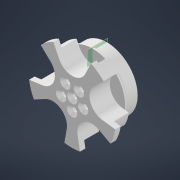
# Autodesk Inventor part: tire cap
Saved by Autodesk Inventor 2022 (Build 260153000, 153)
## iProperties
Created: 2023-02-07
Part Number: tire cap
Material: Типовые
Document SubType Name: Modeling
Designer: akapu
Density: 1 g/cm^3
Appearance: По умолчанию
Author: akapu
Autodesk Inventor part; units mm, degrees
ref_plane "YZ Plane" through (0, 0, 0) normal (1, 0, 0) x (0, 1, 0)
ref_plane "XZ Plane" through (0, 0, 0) normal (0, 1, 0) x (-1, 0, 0)
sketch "Эскиз1" plane through (0, 0, 0) normal (0, 0, 1) x (1, 0, 0)
  circle A0 centre (-27.3933, 9.5988) radius 21.25 projected
  circle A1 centre (-27.3933, 9.5988) radius 18.75 projected
  point P0 (0, 0)
ref_plane "РабПлоскость1" through (-34.9651, 34.6315, 13) normal (0, 0, 1) x (1, 0, 0)
extrude "Выдавливание1" add sketch "Эскиз1" along normal up to surface (13 mm away) contours A0 | A1
ref_plane "РабПлоскость3" through (-27.3933, 9.5988, 13) normal (-1, 0, 0) x (0, -1, 0)
sketch "Эскиз3" plane through (-27.3933, 9.5988, 13) normal (-1, 0, 0) x (0, -1, 0)
  line L0 (-22.45, -4.27) -> (-21.25, -5.47)
  line L1 (-22.45, -3.07) -> (-22.45, -4.27)
  line L2 (30, -3.07) -> (-30, -3.07) projected
  line L3 (30, -3.07) -> (-30, -3.07) projected
  line L4 (-21.25, 0) -> (21.25, 0) projected
  line L5 (-21.25, 0) -> (-30, 0)
  line L6 (-30, 0) -> (-30, -3.07)
  line L7 (-30, -3.07) -> (-21.25, -3.07)
  line L8 (-21.25, -3.07) -> (-21.25, 0)
  line L9 (0, 0) -> (0, -13)
  line L10 (21.25, -13) -> (-21.25, -13) projected
  line L11 (-21.25, -13) -> (-21.25, 0) projected
  line L12 (0, 0) -> (-30, 0)
  line L13 (-30, 0) -> (-30, 11)
  line L14 (-30, 11) -> (0, 11)
  line L15 (0, 11) -> (0, 0)
  line L16 (-25.52, 6.93) -> (-25.52, -23)
  line L17 (-25.32, 6.93) -> (-25.32, -23)
  line L18 (-25.32, 6.93) -> (-25.32, 11)
  line L19 (-25.32, 6.93) -> (-30, 6.93)
  line L20 (-25.32, 7.23) -> (-30, 7.23)
  point P0 (9.5988, -13)
  point P1 (-21.25, -3.07)
  point P2 (-25.32, -3.07)
  dimension "d21" = 11
  dimension "d25" = 0.2
  dimension "d26" = 0.3
  constraints: 32 end point, 6 parallel, 4 perpendicular, 2 horizontal, 2 midpoint, 2 point on line, 2 vertical, 6 other
  measures "d21" distance of L12.end L13.end
  measures "d25" distance between parallel lines of L16 L17
  measures "d26" distance between parallel lines of L19 L20
revolve "Вращение1" add sketch "Эскиз3" angle 360 about axis through (-27.3933, 9.5988, 13) along (0, 0, -1) contours L1 L2 L11 L0 | L2 L17 L5 L8 | L5 L17 L18 L14 L15 L4 | L20 L13 L14 L18
sketch "Эскиз5" plane through (-27.3933, 9.5988, 24) normal (0, 0, 1) x (1, 0, 0)
  circle A0 centre (0, 0) radius 22.45 projected
  line L0 (-30.0943, 4.3007) -> (-34.526, 5.7406) projected
  arc A1 (-34.526, 5.7406) -> (-24.5579, -24.9382) centre (0, 0) ccw projected
  line L1 (-24.5579, -24.9382) -> (-21.8189, -21.1683) projected
  arc A2 (-21.8189, -21.1683) -> (-13.3898, -27.2924) centre (0, 0) ccw projected
  line L2 (-13.3898, -27.2924) -> (-16.1288, -31.0622) projected
  arc A3 (-16.1288, -31.0622) -> (16.1288, -31.0622) centre (0, 0) ccw projected
  line L3 (16.1288, -31.0622) -> (13.3898, -27.2924) projected
  arc A4 (13.3898, -27.2924) -> (21.8189, -21.1683) centre (0, 0) ccw projected
  line L4 (21.8189, -21.1683) -> (24.5579, -24.9382) projected
  arc A5 (24.5579, -24.9382) -> (34.526, 5.7406) centre (0, 0) ccw projected
  line L5 (34.526, 5.7406) -> (30.0943, 4.3007) projected
  arc A6 (30.0943, 4.3007) -> (26.8746, 14.2096) centre (0, 0) ccw projected
  line L6 (26.8746, 14.2096) -> (31.3064, 15.6496) projected
  arc A7 (31.3064, 15.6496) -> (5.2094, 34.6101) centre (0, 0) ccw projected
  line L7 (5.2094, 34.6101) -> (5.2094, 29.9503) projected
  arc A8 (5.2094, 29.9503) -> (-5.2094, 29.9503) centre (0, 0) ccw projected
  line L8 (-5.2094, 29.9503) -> (-5.2094, 34.6101) projected
  arc A9 (-5.2094, 34.6101) -> (-31.3064, 15.6496) centre (0, 0) ccw projected
  line L9 (-31.3064, 15.6496) -> (-26.8746, 14.2096) projected
  arc A10 (-26.8746, 14.2096) -> (-30.0943, 4.3007) centre (0, 0) ccw projected
  line L10 (3.8059, -20.9064) -> (6.2685, -34.4341) projected
  line L11 (18.7071, -10.0801) -> (30.8117, -16.6024) projected
  line L12 (21.0593, -2.8408) -> (34.6858, -4.679) projected
  line L13 (15.3675, 14.6766) -> (25.3112, 24.1732) projected
  line L14 (9.2094, 19.1507) -> (15.1685, 31.5423) projected
  line L15 (-9.2094, 19.1507) -> (-15.1685, 31.5423) projected
  line L16 (-15.3675, 14.6766) -> (-25.3112, 24.1732) projected
  line L17 (-21.0593, -2.8408) -> (-34.6858, -4.679) projected
  line L18 (-18.7071, -10.0801) -> (-30.8117, -16.6024) projected
  line L19 (-3.8059, -20.9064) -> (-6.2685, -34.4341) projected
  circle A11 centre (0, 0) radius 21.25 projected
  line L20 (-9.2094, 19.1507) -> (-9.0121, 18.7403)
  line L21 (9.0121, 18.7403) -> (9.2094, 19.1507)
  line L22 (15.3675, 14.6766) -> (15.0382, 14.3621)
  line L23 (21.0593, -2.8408) -> (20.608, -2.7799)
  line L24 (18.7071, -10.0801) -> (18.3062, -9.864)
  line L25 (3.8059, -20.9064) -> (3.7243, -20.4584)
  line L26 (-3.8059, -20.9064) -> (-3.7243, -20.4584)
  line L27 (-18.7071, -10.0801) -> (-18.3062, -9.864)
  line L28 (-21.0593, -2.8408) -> (-20.608, -2.7799)
  line L29 (-15.3675, 14.6766) -> (-15.0382, 14.3621)
  arc A12 (-20.608, -2.7799) -> (-15.0382, 14.3621) centre (-21.9448, 7.1303) ccw
  arc A13 (-9.0121, 18.7403) -> (9.0121, 18.7403) centre (0, 23.0741) ccw
  arc A14 (15.0382, 14.3621) -> (20.608, -2.7799) centre (21.9448, 7.1303) ccw
  arc A15 (18.3062, -9.864) -> (3.7243, -20.4584) centre (13.5626, -18.6674) ccw
  arc A16 (-3.7243, -20.4584) -> (-18.3062, -9.864) centre (-13.5626, -18.6674) ccw
  point P0 (27.3933, -9.5988)
  dimension "d22" = 10
  constraints: 20 end point, 10 point on circle, 10 point on line, 10 tangent, 5 centre point, 4 equal radius, 1 other
  measures "d22" radius of A12
extrude "Выдавливание3" cut sketch "Эскиз5" against normal up to surface (14.07 mm away) contours A0 L12 A11 L13 | A0 L13 A7 L6 A6 L5 A5 L12 | L14 A11 L15 A0 | A0 L15 A9 L8 A8 L7 A7 L14 | A11 L23 A14 L22 | L11 A5 L4 A4 L3 A3 L10 A0 | A0 L10 A11 L11 | L21 A13 L20 A11 | A11 L25 A15 L24 | L16 A11 L17 A0 | A0 L17 A1 L0 A10 L9 A9 L16 | L19 A3 L2 A2 L1 A1 L18 A0 | A0 L18 A11 L19 | L29 A12 L28 A11 | A11 L27 A16 L26
sketch "Эскиз6" plane through (-27.3933, 9.5988, 13) normal (-1, 0, 0) x (0, -1, 0)
  line L0 (16.6287, -10.8787) -> (-16.6287, -10.8787) projected
  line L1 (-21.25, -13) -> (21.25, -13) projected
  line L2 (-18.75, -13) -> (-16.6287, -10.8787)
  line L3 (18.75, -13) -> (16.6287, -10.8787)
  line L4 (21.25, -13) -> (-21.25, -13) projected
  line L5 (-21.25, -13) -> (-19.25, -13)
  line L6 (-19.25, -13) -> (-17.1287, -10.8787)
  line L7 (0, -10.8787) -> (0, -10.3787)
  line L8 (0, -10.3787) -> (-16.6287, -10.3787)
  line L9 (-16.6287, -10.3787) -> (-17.1287, -10.8787)
  line L10 (0, -10.3787) -> (0, -13)
  line L11 (0, -13) -> (-19.25, -13)
  line L12 (-19.25, -13) -> (-19.25, -10.1)
  line L13 (-19.25, -10.1) -> (0, -10.1)
  line L14 (0, -10.3787) -> (0, -10.1)
  point P0 (20.25, -13)
  point P1 (-19.25, -13)
  dimension "d29" = 2
  dimension "d30" = 135
  dimension "d31" = 0.5
  dimension "d44" = 2.9
  constraints: 24 end point, 3 perpendicular, 2 midpoint, 2 vertical, 1 parallel, 1 point on line, 6 other
  measures "d29" distance of L1.start L5.end
  measures "d30" angle of L6 L5
  measures "d31" distance of L7.start L7.end
  measures "d44" distance of L5.end L12.end
revolve "Вращение2" cut sketch "Эскиз6" angle 360 about axis through (-27.3933, 9.5988, 2.6213) along (0, 0, -1) contours L10 L1 L2 L0 | L0 L2 L1 L6 L9 L8 L7 | L8 L9 L6 L12 L13 L14
sketch "Эскиз7" plane through (-27.3933, 32.6729, 24) normal (0, 0, 1) x (1, 0, 0)
  circle A0 centre (0, -23.0741) radius 22.45 projected
  circle A1 centre (0, -23.0741) radius 1.6
  line L0 (0, -23.0741) -> (0, -31.0741)
  circle A2 centre (0, -31.0741) radius 1.6
  circle A3 centre (7.6085, -25.5463) radius 1.6
  circle A4 centre (4.7023, -16.602) radius 1.6
  circle A5 centre (-4.7023, -16.602) radius 1.6
  circle A6 centre (-7.6085, -25.5463) radius 1.6
  point P0 (27.3933, -32.6729)
  dimension "d33" = 3.2
  dimension "d34" = 8
  dimension "d37" = 360
  constraints: 6 centre point, 2 coincident, 2 end point, 1 vertical, 11 other
  measures "d33" diameter of A1
  measures "d34" distance of L0.start L0.end
extrude "Выдавливание4" cut sketch "Эскиз7" against normal blind 30 contours A1 | A2 | A3 | A4 | A5 | A6
chamfer "Фаска1" distance 2 angle 45 6 edges at (-28.9933, 1.5988, 24) (-36.6017, 7.1266, 24) (-33.6955, 16.0709, 24) (-28.9933, 9.5988, 24) (-24.291, 16.0709, 24) (-21.3848, 7.1266, 24)
